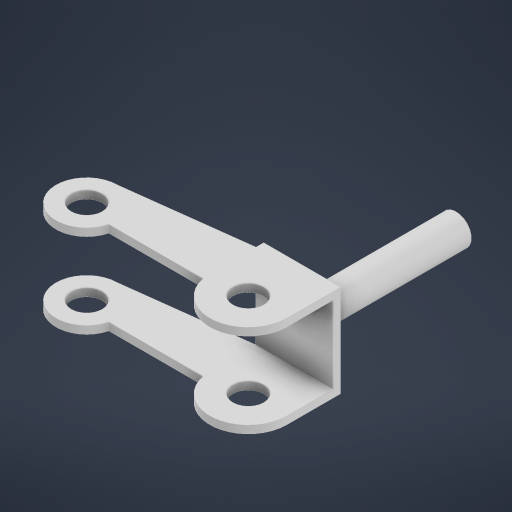
# Autodesk Inventor part: Langbektang houder
Saved by Autodesk Inventor 2023.2 (Build 272271000, 271)
## iProperties
Created: 2020-09-09
Part Number: Langbektang houder
Material: Generic
Document SubType Name: Modeling
Designer: nathan.bollaert
Density: 1 g/cm^3
Appearance: Default
Mass: 0.779151 g
Surface Area: 15.1503 cm^2
Volume: 0.779151 cm^3
Author: nathan.bollaert
Autodesk Inventor part; units mm, degrees
ref_plane "YZ Plane" through (0, 0, 0) normal (1, 0, 0) x (0, 1, 0)
ref_plane "XZ Plane" through (0, 0, 0) normal (0, 1, 0) x (-1, 0, 0)
ref_plane "XY Plane" through (0, 0, 0) normal (0, 0, 1) x (1, 0, 0)
sketch "Sketch1" plane through (0, 0, 0) normal (0, 1, 0) x (-1, 0, 0)
  line L0 (0, -12) -> (10, -12)
  line L1 (10, -12) -> (10, -5)
  line L2 (0, -5) -> (0, -12)
  arc A0 (10, -5) -> (0, -5) centre (5, -5) ccw
  circle A1 centre (5, -5) radius 2
  circle A2 centre (26, -5) radius 2
  line L3 (10, -4) -> (22, -4)
  line L4 (10, -12) -> (10, -11)
  line L5 (26, -9) -> (10, -11)
  arc A3 (26, -9) -> (22, -5) centre (26, -5) ccw
  line L6 (10, -4) -> (9.899, -4)
  line L7 (22, -4) -> (22.127, -4)
  point P0 (0, 0)
  point P1 (0, 0)
  point P2 (9.9495, -4)
  point P3 (5, 0)
  dimension "d269" = 4
  dimension "d270" = 12
  dimension "d271" = 1
  dimension "d272" = 4
  dimension "d273" = 4
  dimension "d274" = -1
  dimension "d275" = -1
  dimension "d278" = 7
  dimension "d279" = 10
  dimension "d280" = 5
  dimension "d282" = 4
  dimension "d284" = 5
  dimension "d286" = 5
  dimension "d287" = 4
  constraints: 16 end point, 7 point on circle, 4 centre point, 4 coincident, 4 horizontal, 2 vertical alignment, 1 midpoint, 1 perpendicular, 1 point on line, 1 tangent
  measures "d269" diameter of A1
  measures "d270" distance of L3.start L3.end
  measures "d271" distance of L1.start L5.end
  measures "d272" diameter of A2
  measures "d273" radius of A3
  measures "d274" vertical distance of L6.end L1.end
  measures "d275" vertical distance of L7.end A3.end
  measures "d278" distance of L2.start L0.start
  measures "d279" distance of L0.start L1.start
  measures "d280" radius of A0
  measures "d282" horizontal distance of L5.start A3.end
  measures "d284" distance of point (0, 0) L2.start
  measures "d286" distance of point (0, 0) point (5, 0)
  measures "d287" horizontal distance of A2.centre L3.end
extrude "Extrusion1" add sketch "Sketch1" along normal blind 1
sketch "Sketch2" plane through (0, 1, 0) normal (0, 1, 0) x (1, 0, 0)
  line L0 (0, 12) -> (-10, 12) projected
  line L1 (0, 12) -> (-10, 12)
  line L2 (-10, 12) -> (-10, 11)
  line L3 (-10, 11) -> (0, 11)
  line L4 (0, 11) -> (0, 12)
  point P0 (0, 0)
  dimension "d288" = 1
  constraints: 8 end point, 3 parallel, 1 horizontal, 1 perpendicular
  measures "d288" distance of L3.end L0.start
extrude "Extrusion2" add sketch "Sketch2" along normal blind 10
sketch "Sketch3" plane through (0, 11, 0) normal (0, 1, 0) x (1, 0, 0)
  line L0 (0, 5) -> (0, 12) projected
  line L1 (0, 12) -> (-10, 12)
  line L2 (-10, 12) -> (-10, 11)
  line L3 (0, 11) -> (0, 12)
  arc A0 (-9.899, 4) -> (0, 5) centre (-5, 5) ccw projected
  line L4 (0, 11) -> (0, 5)
  line L5 (-22.127, 4) -> (-9.899, 4) projected
  arc A1 (-9.899, 4) -> (0, 5) centre (-5, 5) ccw
  arc A2 (-26, 9) -> (-22.127, 4) centre (-26, 5) ccw projected
  line L6 (-9.899, 4) -> (-22.127, 4)
  line L7 (-10, 11) -> (-26, 9) projected
  line L8 (-10, 11) -> (-26, 9)
  circle A3 centre (-5, 5) radius 2
  circle A4 centre (-26, 5) radius 2
  arc A5 (-26, 9) -> (-22.127, 4) centre (-26, 5) ccw
  dimension "d291" = 4
  dimension "d294" = 4
  dimension "d295" = 4
  constraints: 12 end point, 4 centre point, 4 point on circle, 2 coincident, 2 equal length, 2 horizontal, 2 tangent, 1 concentric, 1 perpendicular, 1 vertical
  measures "d291" diameter of A4
  measures "d294" diameter of A3
  measures "d295" radius of A5
extrude "Extrusion3" add sketch "Sketch3" along normal blind 1
sketch "Sketch4" plane through (0, 0, -12) normal (0, 0, -1) x (-1, 0, 0)
  circle A0 centre (5, 6) radius 2
  line L0 (0, 0) -> (10, 0) projected
  line L1 (0, 0) -> (0, 12) projected
  dimension "d269" = 4
  dimension "d270" = 12
  dimension "d271" = 1
  dimension "d272" = 4
  dimension "d273" = 4
  dimension "d274" = -1
  dimension "d275" = -1
  dimension "d278" = 7
  dimension "d279" = 10
  dimension "d280" = 5
  dimension "d282" = 4
  dimension "d284" = 5
  dimension "d286" = 5
  dimension "d287" = 4
  dimension "d296" = 4
  dimension "d297" = 6
  dimension "d298" = 5
  constraints: 1 centre point
  measures "d296" diameter of A0
  measures "d297" distance from line of L0 A0.centre
  measures "d298" distance from line of L1 A0.centre
extrude "Extrusion4" add sketch "Sketch4" along normal blind 20
body "Solid5"
